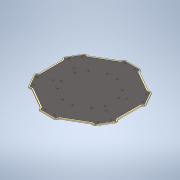
# Autodesk Inventor part: FRAME BAWAH
Saved by Autodesk Inventor 2020.2 (Build 242310000, 310)
## iProperties
Created: 2020-03-27
Part Number: FRAME BAWAH
Material: Generic
Document SubType Name: Modeling
Designer: Muhyidin
Density: 1 g/cm^3
Appearance: Carbon Fiber
Author: Muhyidin
Autodesk Inventor part; units mm, degrees
ref_plane "YZ Plane" through (0, 0, 0) normal (1, 0, 0) x (0, 1, 0)
ref_plane "XZ Plane" through (0, 0, 0) normal (0, 1, 0) x (-1, 0, 0)
ref_plane "XY Plane" through (0, 0, 0) normal (0, 0, 1) x (1, 0, 0)
sketch "Sketch1" plane through (0, 0, 0) normal (0, 1, 0) x (-1, 0, 0)
  circle A0 centre (15.3999, -131.0001) radius 1.6
  circle A1 centre (-15.4001, -131) radius 1.6
  line L0 (-83.9102, 30.6632) -> (-53.9102, 30.6632) construction
  line L1 (-76.2102, -44) -> (-51.2102, -44) construction
  line L2 (25, -145) -> (60, -145) construction
  line L3 (0, -138) -> (25, -138)
  line L4 (0, -138) -> (25, -138) construction
  line L5 (0, -138) -> (-25, -138)
  line L6 (0, -138) -> (25, -138) construction
  line L7 (15.4, -138) -> (22.4, -138) construction
  line L8 (-15.4, -138.0001) -> (-8.4, -138.0001) construction
  line L9 (-25, -138) -> (4.9988, -138) construction
  line L10 (-92.0115, -90.6506) -> (-87.0115, -90.6506) construction
  line L11 (-25, -138) -> (-5.0008, -138) construction
  line L12 (-25, -138) -> (-28.4202, -128.6031)
  line L13 (-25, -138) -> (-15, -138) construction
  line L14 (25, -138) -> (28.4201, -128.6031)
  line L15 (132.0114, -47.3494) -> (125.5835, -39.689)
  line L16 (107.0114, -90.6507) -> (97.1633, -88.9142)
  line L17 (111.8115, -82.3369) -> (115.3115, -76.2747) construction
  line L18 (107.0114, -90.6507) -> (117.011, -73.3308) construction
  line L19 (119.5114, -69) -> (107.0114, -90.6507)
  line L20 (107.0114, -90.6507) -> (122.0108, -64.6709) construction
  line L21 (119.5114, -69) -> (132.0114, -47.3494)
  line L22 (119.5114, -69) -> (132.0114, -47.3494) construction
  line L23 (119.5114, -69) -> (132.0114, -47.3494) construction
  circle A2 centre (121.1493, -52.1634) radius 1.6
  circle A3 centre (105.7492, -78.8369) radius 1.6
  line L24 (107.0114, 90.6505) -> (97.1634, 88.914)
  line L25 (132.0114, 47.3493) -> (125.5835, 39.6888)
  line L26 (127.2115, 55.6631) -> (123.7115, 61.7253) construction
  line L27 (132.0114, 47.3493) -> (122.0118, 64.6691) construction
  line L28 (119.5114, 68.9999) -> (132.0114, 47.3493)
  line L29 (132.0114, 47.3493) -> (117.012, 73.329) construction
  line L30 (119.5114, 68.9999) -> (107.0114, 90.6505)
  line L31 (119.5114, 68.9999) -> (107.0114, 90.6505) construction
  line L32 (119.5114, 68.9999) -> (107.0114, 90.6505) construction
  circle A4 centre (105.7494, 78.8366) radius 1.6
  circle A5 centre (121.1493, 52.163) radius 1.6
  line L33 (-25.0001, 137.9998) -> (-28.4202, 128.6029)
  line L34 (24.9999, 137.9998) -> (28.4202, 128.6029)
  line L35 (15.4, 137.9999) -> (8.4, 137.9999) construction
  line L36 (24.9999, 137.9998) -> (5.0007, 137.9998) construction
  line L37 (-0.0001, 137.9998) -> (24.9999, 137.9998)
  line L38 (24.9999, 137.9998) -> (-4.9989, 137.9998) construction
  line L39 (-0.0001, 137.9998) -> (-25.0001, 137.9998)
  line L40 (-0.0001, 137.9998) -> (-25.0001, 137.9998) construction
  line L41 (-0.0001, 137.9998) -> (-25.0001, 137.9998) construction
  circle A6 centre (-15.3999, 130.9999) radius 1.6
  circle A7 centre (15.4, 130.9999) radius 1.6
  line L42 (-132.0115, 47.3492) -> (-125.5836, 39.6889)
  line L43 (-107.0115, 90.6505) -> (-97.1634, 88.914)
  line L44 (-111.8115, 82.3367) -> (-115.3115, 76.2745) construction
  line L45 (-107.0115, 90.6505) -> (-117.0111, 73.3307) construction
  line L46 (-119.5115, 68.9999) -> (-107.0115, 90.6505)
  line L47 (-107.0115, 90.6505) -> (-122.0109, 64.6707) construction
  line L48 (-119.5115, 68.9999) -> (-132.0115, 47.3492)
  line L49 (-119.5115, 68.9999) -> (-132.0115, 47.3492) construction
  line L50 (-119.5115, 68.9999) -> (-132.0115, 47.3492) construction
  circle A8 centre (-121.1493, 52.1632) radius 1.6
  circle A9 centre (-105.7493, 78.8367) radius 1.6
  line L51 (-107.0114, -90.6507) -> (-97.1634, -88.9142)
  line L52 (-132.0114, -47.3494) -> (-125.5836, -39.689)
  line L53 (-127.2115, -55.6633) -> (-123.7115, -61.7255) construction
  line L54 (-132.0114, -47.3494) -> (-122.0118, -64.6693) construction
  line L55 (-119.5114, -69.0001) -> (-132.0114, -47.3494)
  line L56 (-132.0114, -47.3494) -> (-117.012, -73.3292) construction
  line L57 (-119.5114, -69.0001) -> (-107.0114, -90.6507)
  line L58 (-119.5114, -69.0001) -> (-107.0114, -90.6507) construction
  line L59 (-119.5114, -69.0001) -> (-107.0114, -90.6507) construction
  circle A10 centre (-105.7494, -78.8368) radius 1.6
  circle A11 centre (-121.1493, -52.1632) radius 1.6
  line L60 (-28.4202, -128.6031) -> (-97.1634, -88.9142)
  line L61 (-15.4, -131) -> (42.1, -131) construction
  line L62 (0, -138) -> (0, -141)
  line L63 (0, -138) -> (3, -138) construction
  line L64 (-25, -138) -> (-22, -138) construction
  line L65 (-25, -138) -> (-20, -138) construction
  line L66 (0, -141) -> (-27.5173, -141)
  line L67 (0, -141) -> (27.5173, -141) construction
  line L68 (-27.5173, -141) -> (-13.8071, -141) construction
  line L69 (-28.4202, -128.6031) -> (-34.2721, -128.6031)
  line L70 (-28.4202, -128.6031) -> (-22.5683, -128.6031) construction
  line L71 (-107.0114, -90.6507) -> (-104.0114, -90.6507) construction
  line L72 (-27.5173, -141) -> (-30.9375, -131.6031)
  line L73 (-27.5173, -141) -> (-17.5173, -141) construction
  line L74 (0, -141) -> (27.5173, -141)
  line L75 (27.5173, -141) -> (13.8071, -141) construction
  line L76 (27.5173, -141) -> (30.9375, -131.6031)
  line L77 (108.3508, -94.3307) -> (98.5028, -92.5942)
  line L78 (122.1095, -70.5) -> (108.3508, -94.3307)
  line L79 (122.1095, -70.5) -> (135.8681, -46.6693) construction
  line L80 (122.1095, -70.5) -> (135.8681, -46.6693)
  line L81 (135.8681, -46.6693) -> (129.4403, -39.0089)
  line L82 (135.8681, 46.6692) -> (129.4402, 39.0088)
  line L83 (122.1095, 70.4999) -> (135.8681, 46.6692)
  line L84 (122.1095, 70.4999) -> (108.3508, 94.3306) construction
  line L85 (122.1095, 70.4999) -> (108.3508, 94.3306)
  line L86 (108.3508, 94.3306) -> (98.5027, 92.5941)
  line L87 (27.5172, 140.9998) -> (30.9374, 131.6029)
  line L88 (-0.0001, 140.9998) -> (27.5172, 140.9998)
  line L89 (-0.0001, 140.9998) -> (-27.5173, 140.9998) construction
  line L90 (-0.0001, 140.9998) -> (-27.5173, 140.9998)
  line L91 (-27.5173, 140.9998) -> (-30.9376, 131.6029)
  line L92 (-108.3509, 94.3305) -> (-98.5028, 92.5941)
  line L93 (-122.1095, 70.4999) -> (-108.3509, 94.3305)
  line L94 (-122.1095, 70.4999) -> (-135.8682, 46.6692) construction
  line L95 (-122.1095, 70.4999) -> (-135.8682, 46.6692)
  line L96 (-135.8682, 46.6692) -> (-129.4403, 39.0087)
  line L97 (-135.8682, -46.6694) -> (-129.4403, -39.0089)
  line L98 (-122.1095, -70.5001) -> (-135.8682, -46.6694)
  line L99 (-122.1095, -70.5001) -> (-108.3509, -94.3307) construction
  line L100 (-122.1095, -70.5001) -> (-108.3509, -94.3307)
  line L101 (-108.3509, -94.3307) -> (-98.5028, -92.5943)
  line L102 (-30.9375, -131.6031) -> (-98.5028, -92.5943)
  line L103 (98.5028, -92.5942) -> (30.9375, -131.6031)
  line L104 (129.4402, 39.0088) -> (129.4403, -39.0089)
  line L105 (30.9374, 131.6029) -> (98.5027, 92.5941)
  line L106 (-98.5028, 92.5941) -> (-30.9376, 131.6029)
  line L107 (-129.4403, -39.0089) -> (-129.4403, 39.0087)
  line L108 (-15.4, -131) -> (42.1, -131) construction
  line L109 (15.3999, -73.5001) -> (15.9999, -73.5001)
  line L110 (15.3999, -73.5001) -> (15.9999, -73.5001) construction
  circle A12 centre (15.9999, -73.5001) radius 1.65
  line L111 (-15.4, -73.5) -> (-16.036, -73.5)
  circle A13 centre (-16.0361, -73.5) radius 1.65
  circle A14 centre (55.6348, -50.6377) radius 1.65
  circle A15 centre (71.6528, -22.8937) radius 1.65
  circle A16 centre (71.6708, 22.8623) radius 1.65
  circle A17 centre (55.6529, 50.6063) radius 1.65
  circle A18 centre (16.036, 73.4999) radius 1.65
  circle A19 centre (-15.9999, 73.4999) radius 1.65
  circle A20 centre (-55.6348, 50.6375) radius 1.65
  circle A21 centre (-71.6529, 22.8936) radius 1.65
  circle A22 centre (-71.6709, -22.8624) radius 1.65
  circle A23 centre (-55.6529, -50.6064) radius 1.65
  line L112 (129.4403, -11) -> (134.4403, -11) construction
  line L113 (28.4201, -128.6031) -> (97.1633, -88.9142)
  line L114 (97.1634, 88.914) -> (28.4202, 128.6029)
  line L115 (-28.4202, 128.6029) -> (-97.1634, 88.914)
  line L116 (125.5835, -39.689) -> (125.5835, 39.6888)
  line L117 (-125.5836, -39.689) -> (-125.5836, 39.6889)
  line L118 (0, -0.0001) -> (87.249, -0.0001)
  line L119 (0, -0.0001) -> (87.249, -0.0001) construction
  line L120 (0, -0.0001) -> (-87.249, -0.0001)
  line L121 (0, -0.0001) -> (-87.249, -0.0001) construction
  line L122 (87.249, -0.0001) -> (87.249, -34.0851)
  line L123 (87.249, -0.0001) -> (121.334, -0.0001) construction
  line L124 (87.249, -0.0001) -> (87.249, 34.0849)
  line L125 (-87.249, -0.0001) -> (-87.249, -34.0851)
  line L126 (-87.249, -0.0001) -> (-87.249, 34.0849)
  circle A24 centre (87.249, -34.0851) radius 1.27
  circle A25 centre (87.249, 34.0849) radius 1.27
  circle A26 centre (-87.249, 34.0849) radius 1.27
  circle A27 centre (-87.249, -34.0851) radius 1.27
  dimension "d427" = 3.2
  dimension "d428" = 3.2
  dimension "d625" = 0
  dimension "d627" = 180
  dimension "d646" = 10
  dimension "d647" = 110
  dimension "d650" = 360
  dimension "d722" = 3
  dimension "d723" = 90
  dimension "d729" = 180
  dimension "d731" = 180
  dimension "d735" = 10
  dimension "d736" = 110
  dimension "d739" = 360
  dimension "d743" = 360
  dimension "d841" = 0.6
  dimension "d842" = 0
  dimension "d856" = 0.636
  dimension "d872" = 360
  dimension "d1043" = 87.249
  dimension "d1044" = 0
  dimension "d1045" = 34.085
  dimension "d1046" = 90
  dimension "d1047" = 2.54
  dimension "d1056" = 2.54
  dimension "d1065" = 2.54
  dimension "d1074" = 2.54
  constraints: 254 end point, 29 horizontal, 28 centre point, 10 equal length, 4 symmetric about line, 2 perpendicular, 2 vertical, 1 coincident, 1 point on line, 250 other
  measures "d427" diameter of A0
  measures "d428" diameter of A1
  measures "d625" distance between parallel lines of L3 L4
  measures "d627" angle of L5 L6
  measures "d646" distance of L5.end L12.end
  measures "d647" angle of L13 L12
  measures "d722" distance of L3.start L62.end
  measures "d723" angle of L62 L63
  measures "d729" angle of L66 L67
  measures "d731" angle of L69 L70
  measures "d735" distance of L66.end L72.end
  measures "d736" angle of L73 L72
  measures "d841" distance of L109.start L109.end
  measures "d842" distance between parallel lines of L109 L110
  measures "d856" distance of L111.start L111.end
  measures "d1043" distance of L118.start L118.end
  measures "d1044" distance between parallel lines of L118 L119
  measures "d1045" distance of L119.end L122.end
  measures "d1046" angle of L122 L123
  measures "d1047" diameter of A24
  measures "d1056" diameter of A25
  measures "d1065" diameter of A26
  measures "d1074" diameter of A27
extrude "Extrusion11" add sketch "Sketch1" along normal blind 3 contours L5 L12 L60 L51 L57 L55 L52 L117 L42 L48 L46 L43 L115 L33 L39 L37 L34 L114 L24 L30 L28 L25 L116 L15 L21 L19 L16 L113 L14 L3
sketch "Sketch3" plane through (0, 3, 0) normal (0, 1, 0) x (1, 0, 0)
  circle A0 centre (15.3999, -131.0001) radius 1.6
  circle A1 centre (-15.4001, -131) radius 1.6
  line L0 (-83.9102, 30.6632) -> (-53.9102, 30.6632) construction
  line L1 (-76.2102, -44) -> (-51.2102, -44) construction
  line L2 (25, -145) -> (60, -145) construction
  line L3 (0, -138) -> (25, -138)
  line L4 (0, -138) -> (25, -138) construction
  line L5 (0, -138) -> (-25, -138)
  line L6 (0, -138) -> (25, -138) construction
  line L7 (15.4, -138) -> (22.4, -138) construction
  line L8 (-15.4, -138.0001) -> (-8.4, -138.0001) construction
  line L9 (-25, -138) -> (4.9988, -138) construction
  line L10 (-92.0115, -90.6506) -> (-87.0115, -90.6506) construction
  line L11 (-25, -138) -> (-5.0008, -138) construction
  line L12 (-25, -138) -> (-28.4202, -128.6031)
  line L13 (-25, -138) -> (-15, -138) construction
  line L14 (25, -138) -> (28.4201, -128.6031)
  line L15 (132.0114, -47.3494) -> (125.5835, -39.689)
  line L16 (107.0114, -90.6507) -> (97.1633, -88.9142)
  line L17 (111.8115, -82.3369) -> (115.3115, -76.2747) construction
  line L18 (107.0114, -90.6507) -> (117.011, -73.3308) construction
  line L19 (119.5114, -69) -> (107.0114, -90.6507)
  line L20 (107.0114, -90.6507) -> (122.0108, -64.6709) construction
  line L21 (119.5114, -69) -> (132.0114, -47.3494)
  line L22 (119.5114, -69) -> (132.0114, -47.3494) construction
  line L23 (119.5114, -69) -> (132.0114, -47.3494) construction
  circle A2 centre (121.1493, -52.1634) radius 1.6
  circle A3 centre (105.7492, -78.8369) radius 1.6
  line L24 (107.0114, 90.6505) -> (97.1634, 88.914)
  line L25 (132.0114, 47.3493) -> (125.5835, 39.6888)
  line L26 (127.2115, 55.6631) -> (123.7115, 61.7253) construction
  line L27 (132.0114, 47.3493) -> (122.0118, 64.6691) construction
  line L28 (119.5114, 68.9999) -> (132.0114, 47.3493)
  line L29 (132.0114, 47.3493) -> (117.012, 73.329) construction
  line L30 (119.5114, 68.9999) -> (107.0114, 90.6505)
  line L31 (119.5114, 68.9999) -> (107.0114, 90.6505) construction
  line L32 (119.5114, 68.9999) -> (107.0114, 90.6505) construction
  circle A4 centre (105.7494, 78.8366) radius 1.6
  circle A5 centre (121.1493, 52.163) radius 1.6
  line L33 (-25.0001, 137.9998) -> (-28.4202, 128.6029)
  line L34 (24.9999, 137.9998) -> (28.4202, 128.6029)
  line L35 (15.4, 137.9999) -> (8.4, 137.9999) construction
  line L36 (24.9999, 137.9998) -> (5.0007, 137.9998) construction
  line L37 (-0.0001, 137.9998) -> (24.9999, 137.9998)
  line L38 (24.9999, 137.9998) -> (-4.9989, 137.9998) construction
  line L39 (-0.0001, 137.9998) -> (-25.0001, 137.9998)
  line L40 (-0.0001, 137.9998) -> (-25.0001, 137.9998) construction
  line L41 (-0.0001, 137.9998) -> (-25.0001, 137.9998) construction
  circle A6 centre (-15.3999, 130.9999) radius 1.6
  circle A7 centre (15.4, 130.9999) radius 1.6
  line L42 (-132.0115, 47.3492) -> (-125.5836, 39.6889)
  line L43 (-107.0115, 90.6505) -> (-97.1634, 88.914)
  line L44 (-111.8115, 82.3367) -> (-115.3115, 76.2745) construction
  line L45 (-107.0115, 90.6505) -> (-117.0111, 73.3307) construction
  line L46 (-119.5115, 68.9999) -> (-107.0115, 90.6505)
  line L47 (-107.0115, 90.6505) -> (-122.0109, 64.6707) construction
  line L48 (-119.5115, 68.9999) -> (-132.0115, 47.3492)
  line L49 (-119.5115, 68.9999) -> (-132.0115, 47.3492) construction
  line L50 (-119.5115, 68.9999) -> (-132.0115, 47.3492) construction
  circle A8 centre (-121.1493, 52.1632) radius 1.6
  circle A9 centre (-105.7493, 78.8367) radius 1.6
  line L51 (-107.0114, -90.6507) -> (-97.1634, -88.9142)
  line L52 (-132.0114, -47.3494) -> (-125.5836, -39.689)
  line L53 (-127.2115, -55.6633) -> (-123.7115, -61.7255) construction
  line L54 (-132.0114, -47.3494) -> (-122.0118, -64.6693) construction
  line L55 (-119.5114, -69.0001) -> (-132.0114, -47.3494)
  line L56 (-132.0114, -47.3494) -> (-117.012, -73.3292) construction
  line L57 (-119.5114, -69.0001) -> (-107.0114, -90.6507)
  line L58 (-119.5114, -69.0001) -> (-107.0114, -90.6507) construction
  line L59 (-119.5114, -69.0001) -> (-107.0114, -90.6507) construction
  circle A10 centre (-105.7494, -78.8368) radius 1.6
  circle A11 centre (-121.1493, -52.1632) radius 1.6
  line L60 (-28.4202, -128.6031) -> (-97.1634, -88.9142)
  line L61 (-15.4, -131) -> (42.1, -131) construction
  line L62 (0, -138) -> (0, -141)
  line L63 (0, -138) -> (3, -138) construction
  line L64 (-25, -138) -> (-22, -138) construction
  line L65 (-25, -138) -> (-20, -138) construction
  line L66 (0, -141) -> (-27.5173, -141)
  line L67 (0, -141) -> (27.5173, -141) construction
  line L68 (-27.5173, -141) -> (-13.8071, -141) construction
  line L69 (-28.4202, -128.6031) -> (-34.2721, -128.6031)
  line L70 (-28.4202, -128.6031) -> (-22.5683, -128.6031) construction
  line L71 (-107.0114, -90.6507) -> (-104.0114, -90.6507) construction
  line L72 (-27.5173, -141) -> (-30.9375, -131.6031)
  line L73 (-27.5173, -141) -> (-17.5173, -141) construction
  line L74 (0, -141) -> (27.5173, -141)
  line L75 (27.5173, -141) -> (13.8071, -141) construction
  line L76 (27.5173, -141) -> (30.9375, -131.6031)
  line L77 (108.3508, -94.3307) -> (98.5028, -92.5942)
  line L78 (122.1095, -70.5) -> (108.3508, -94.3307)
  line L79 (122.1095, -70.5) -> (135.8681, -46.6693) construction
  line L80 (122.1095, -70.5) -> (135.8681, -46.6693)
  line L81 (135.8681, -46.6693) -> (129.4403, -39.0089)
  line L82 (135.8681, 46.6692) -> (129.4402, 39.0088)
  line L83 (122.1095, 70.4999) -> (135.8681, 46.6692)
  line L84 (122.1095, 70.4999) -> (108.3508, 94.3306) construction
  line L85 (122.1095, 70.4999) -> (108.3508, 94.3306)
  line L86 (108.3508, 94.3306) -> (98.5027, 92.5941)
  line L87 (27.5172, 140.9998) -> (30.9374, 131.6029)
  line L88 (-0.0001, 140.9998) -> (27.5172, 140.9998)
  line L89 (-0.0001, 140.9998) -> (-27.5173, 140.9998) construction
  line L90 (-0.0001, 140.9998) -> (-27.5173, 140.9998)
  line L91 (-27.5173, 140.9998) -> (-30.9376, 131.6029)
  line L92 (-108.3509, 94.3305) -> (-98.5028, 92.5941)
  line L93 (-122.1095, 70.4999) -> (-108.3509, 94.3305)
  line L94 (-122.1095, 70.4999) -> (-135.8682, 46.6692) construction
  line L95 (-122.1095, 70.4999) -> (-135.8682, 46.6692)
  line L96 (-135.8682, 46.6692) -> (-129.4403, 39.0087)
  line L97 (-135.8682, -46.6694) -> (-129.4403, -39.0089)
  line L98 (-122.1095, -70.5001) -> (-135.8682, -46.6694)
  line L99 (-122.1095, -70.5001) -> (-108.3509, -94.3307) construction
  line L100 (-122.1095, -70.5001) -> (-108.3509, -94.3307)
  line L101 (-108.3509, -94.3307) -> (-98.5028, -92.5943)
  line L102 (-30.9375, -131.6031) -> (-98.5028, -92.5943)
  line L103 (98.5028, -92.5942) -> (30.9375, -131.6031)
  line L104 (129.4402, 39.0088) -> (129.4403, -39.0089)
  line L105 (30.9374, 131.6029) -> (98.5027, 92.5941)
  line L106 (-98.5028, 92.5941) -> (-30.9376, 131.6029)
  line L107 (-129.4403, -39.0089) -> (-129.4403, 39.0087)
  line L108 (-15.4, -131) -> (42.1, -131) construction
  line L109 (15.3999, -73.5001) -> (15.9999, -73.5001)
  line L110 (15.3999, -73.5001) -> (15.9999, -73.5001) construction
  circle A12 centre (15.9999, -73.5001) radius 1.65
  line L111 (-15.4, -73.5) -> (-16.036, -73.5)
  circle A13 centre (-16.0361, -73.5) radius 1.65
  circle A14 centre (55.6348, -50.6377) radius 1.65
  circle A15 centre (71.6528, -22.8937) radius 1.65
  circle A16 centre (71.6708, 22.8623) radius 1.65
  circle A17 centre (55.6529, 50.6063) radius 1.65
  circle A18 centre (16.036, 73.4999) radius 1.65
  circle A19 centre (-15.9999, 73.4999) radius 1.65
  circle A20 centre (-55.6348, 50.6375) radius 1.65
  circle A21 centre (-71.6529, 22.8936) radius 1.65
  circle A22 centre (-71.6709, -22.8624) radius 1.65
  circle A23 centre (-55.6529, -50.6064) radius 1.65
  line L112 (129.4403, -11) -> (134.4403, -11) construction
  line L113 (28.4201, -128.6031) -> (97.1633, -88.9142)
  line L114 (97.1634, 88.914) -> (28.4202, 128.6029)
  line L115 (-28.4202, 128.6029) -> (-97.1634, 88.914)
  line L116 (125.5835, -39.689) -> (125.5835, 39.6888)
  line L117 (-125.5836, -39.689) -> (-125.5836, 39.6889)
  line L118 (0, -0.0001) -> (87.249, -0.0001)
  line L119 (0, -0.0001) -> (87.249, -0.0001) construction
  line L120 (0, -0.0001) -> (-87.249, -0.0001) construction
  line L121 (0, -0.0001) -> (-87.249, -0.0001)
  line L122 (87.249, -0.0001) -> (87.249, -34.0851)
  line L123 (87.249, -0.0001) -> (121.334, -0.0001) construction
  line L124 (87.249, -0.0001) -> (87.249, 34.0849)
  line L125 (-87.249, -0.0001) -> (-87.249, -34.0851)
  line L126 (-87.249, -0.0001) -> (-87.249, 34.0849)
  circle A24 centre (87.249, -34.0851) radius 1.27
  circle A25 centre (87.249, 34.0849) radius 1.27
  circle A26 centre (-87.249, 34.0849) radius 1.27
  circle A27 centre (-87.249, -34.0851) radius 1.27
  point P0 (28.4201, -128.6031)
  point P1 (-28.4202, 128.6029)
  point P2 (28.4201, -128.6031)
  point P3 (-28.4202, 128.6029)
  point P4 (-36.5897, -0.0001)
  point P5 (36.5897, -0.0001)
  point P6 (129.4403, -39.0089)
  dimension "d1083" = 3.2
  dimension "d1084" = 3.2
  dimension "d1085" = 0
  dimension "d1086" = 180
  dimension "d1087" = 10
  dimension "d1088" = 110
  dimension "d1089" = 360
  dimension "d1090" = 3
  dimension "d1091" = 90
  dimension "d1092" = 180
  dimension "d1093" = 180
  dimension "d1094" = 10
  dimension "d1095" = 110
  dimension "d1096" = 360
  dimension "d1097" = 360
  dimension "d1098" = 0.6
  dimension "d1099" = 0
  dimension "d1100" = 0.636
  dimension "d1101" = 360
  dimension "d1102" = 87.249
  dimension "d1103" = 0
  dimension "d1104" = 34.085
  dimension "d1105" = 90
  dimension "d1106" = 2.54
  dimension "d1107" = 2.54
  dimension "d1108" = 2.54
  dimension "d1109" = 2.54
  constraints: 254 end point, 29 horizontal, 28 centre point, 10 equal length, 4 symmetric about line, 2 perpendicular, 2 vertical, 1 coincident, 1 point on line, 250 other
  measures "d1083" diameter of A0
  measures "d1084" diameter of A1
  measures "d1085" distance between parallel lines of L3 L4
  measures "d1086" angle of L5 L6
  measures "d1087" distance of L5.end L12.end
  measures "d1088" angle of L13 L12
  measures "d1090" distance of L3.start L62.end
  measures "d1091" angle of L62 L63
  measures "d1092" angle of L66 L67
  measures "d1093" angle of L69 L70
  measures "d1094" distance of L66.end L72.end
  measures "d1095" angle of L73 L72
  measures "d1098" distance of L109.start L109.end
  measures "d1099" distance between parallel lines of L109 L110
  measures "d1100" distance of L111.start L111.end
  measures "d1102" distance of L118.start L118.end
  measures "d1103" distance between parallel lines of L118 L119
  measures "d1104" distance of L119.end L122.end
  measures "d1105" angle of L122 L123
  measures "d1106" diameter of A24
  measures "d1107" diameter of A25
  measures "d1108" diameter of A26
  measures "d1109" diameter of A27
extrude "Extrusion12" add sketch "Sketch3" against normal blind 3 separate body contours L66 L72 L102 L101 L100 L98 L97 L107 L96 L95 L93 L92 L106 L91 L90 L88 L87 L105 L86 L85 L83 L82 L104 L81 L80 L78 L77 L103 L76 L74
fillet "Fillet12" radius 5 24 edges at (98.5028, 1.5, 92.5942) (108.3508, 1.5, 94.3307) (135.8681, 1.5, 46.6693) (129.4403, 1.5, 39.0089) (129.4402, 1.5, -39.0088) (135.8681, 1.5, -46.6692) (108.3508, 1.5, -94.3306) (98.5027, 1.5, -92.5941) (30.9374, 1.5, -131.6029) (27.5172, 1.5, -140.9998) (-30.9376, 1.5, -131.6029) (-27.5173, 1.5, -140.9998) (-98.5028, 1.5, -92.5941) (-108.3509, 1.5, -94.3305) (-135.8682, 1.5, -46.6692) (-129.4403, 1.5, -39.0087) (-129.4403, 1.5, 39.0089) (-135.8682, 1.5, 46.6694) (-108.3509, 1.5, 94.3307) (-98.5028, 1.5, 92.5943) (-30.9375, 1.5, 131.6031) (-27.5173, 1.5, 141) (27.5173, 1.5, 141) (30.9375, 1.5, 131.6031)
body "Solid11"
body "Solid12"
